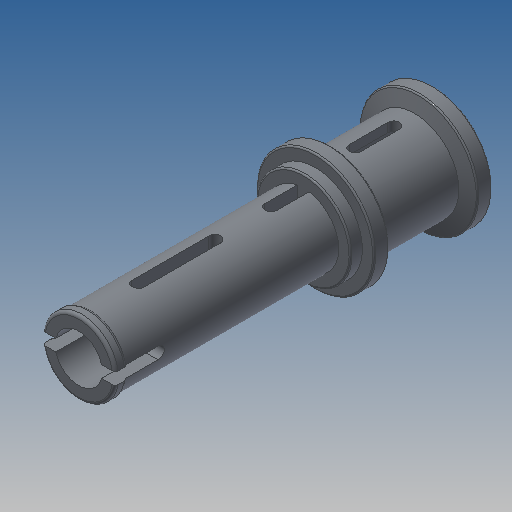
# Autodesk Inventor part: 32054-LtBluishGray
Saved by Autodesk Inventor 2022.2 (Build 262287000, 287)
## iProperties
Created: 2014-06-03
Part Number: 32054-LtBluishGray
Material: ABS Plastic
Document SubType Name: Modeling
Designer: D. Kohfeld
Appearance: LtBluishGray
Density: 1.06 g/cm^3
Mass: 0.348548 g
Surface Area: 8.37071 cm^2
Volume: 0.328818 cm^3
Author: D. Kohfeld
Autodesk Inventor part; units mm, degrees
ref_plane "YZ Plane" through (0, 0, 0) normal (1, 0, 0) x (0, 1, 0)
ref_plane "XZ Plane" through (0, 0, 0) normal (0, 1, 0) x (-1, 0, 0)
ref_plane "XY Plane" through (0, 0, 0) normal (0, 0, 1) x (1, 0, 0)
sketch "Sketch1" plane through (0, 0, 0) normal (0, 1, 0) x (-1, 0, 0)
  line L0 (2.4, 15.2) -> (2.4, 0.8)
  line L1 (3.2, 0.8) -> (2.4, 0.8)
  line L2 (3.2, 0.8) -> (3.2, 0)
  line L3 (3, -6.7321) -> (3, -1.2679)
  line L4 (2.5, 16) -> (2.5, 15.2)
  line L5 (2.5, 16) -> (1.6, 16)
  line L6 (0, -15.68) -> (0, 21.28) projected
  line L7 (2.4, 15.2) -> (2.5, 15.2)
  line L8 (5.28, 0) -> (-3.68, 0) projected
  line L9 (0, -8) -> (4, -8)
  line L10 (4, -8) -> (4, -7)
  line L11 (-0.4, 3) -> (-0.4, 0.8)
  line L12 (0.4, 0.8) -> (0.4, 3)
  arc A0 (0.4, 3) -> (-0.4, 3) centre (0, 3) ccw
  line L13 (-0.4, 12) -> (-0.4, 6.8)
  arc A1 (-0.4, 6.8) -> (0.4, 6.8) centre (0, 6.8) ccw
  line L14 (0.4, 6.8) -> (0.4, 12)
  arc A2 (0.4, 12) -> (-0.4, 12) centre (0, 12) ccw
  line L15 (3.2, 0) -> (4, 0)
  line L16 (4, 0) -> (4, -1)
  line L17 (4, -1) -> (3, -1.2679)
  line L18 (4, -7) -> (3, -6.7321)
  circle A3 centre (0, -8) radius 2.4 construction
  line L19 (-0.4, 0.8) -> (0.4, 0.8)
  line L20 (0.4, -2.7) -> (0.4, -5.3)
  arc A4 (-0.4, -5.3) -> (0.4, -5.3) centre (0, -5.3) ccw
  line L21 (-0.4, -5.3) -> (-0.4, -2.7)
  arc A5 (0.4, -2.7) -> (-0.4, -2.7) centre (0, -2.7) ccw
  line L22 (1.6, 16) -> (1.6, 0)
  line L23 (1.6, 0) -> (0, 0)
  line L24 (0, 0) -> (0, -8)
  point P0 (0.4, -4)
  point P1 (3, -4)
  dimension "d1" = 4.8
  dimension "d2" = 5
  dimension "d6" = 16
  dimension "d7" = 0.8
  dimension "d8" = 6.4
  dimension "d9" = 0.8
  dimension "d14" = 0.8
  dimension "d16" = 6
  dimension "d17" = 0.8
  dimension "d18" = 4
  dimension "d19" = 8
  dimension "d30" = 8
  dimension "d32" = 4.8
  dimension "d33" = 1
  dimension "d35" = 15
  dimension "d36" = 0.6
  dimension "d37" = 3.4
  dimension "d38" = 3.4
  dimension "d46" = 3.2
  constraints: 46 end point, 10 point on circle, 10 tangent, 7 point on line, 6 centre point, 6 parallel, 5 perpendicular, 3 vertical, 2 collinear, 2 equal length, 2 horizontal alignment, 2 midpoint, 1 equal radius, 1 vertical alignment
  measures "d1" diameter of L0 L6
  measures "d2" diameter of L4 L6
  measures "d6" distance between parallel lines of L5 L8
  measures "d7" distance from line of L4.end L5
  measures "d8" diameter of L2 L6
  measures "d9" distance between parallel lines of L1 L8
  measures "d14" diameter of A0
  measures "d17" diameter of A2
  measures "d18" distance from line of A2.centre L5
  measures "d19" distance between parallel lines of L9 L8
  measures "d30" diameter of L10 L6
  measures "d32" diameter of A3
  measures "d33" distance of L9.end L10.end
  measures "d35" angle of L18 L9
  measures "d36" distance edge to line of A3 L3
  measures "d46" diameter of L22 L6
revolve "Revolution1" add sketch "Sketch1" angle 360 about axis through (0, 0, -10) along (0, 0, 1) contours L0 L1 L2 L8 L22 L5 L4 L7 | L8 L16 L17 L3 L18 L10 L9 L6 A4 L20 A5 | A5 L20 A4 L6
fillet "Fillet1" radius 0.2 2 edges at (2.5, 0, 16) (2.5, 0, 15.2)
fillet "Fillet1" radius 0.1 5 edges at (4, 0, 0) (4, 0, -1) (4, 0, -7) (4, 0, -8) (3.2, 0, 0.8)
extrude "Extrusion1" cut sketch "Sketch1" along normal through all both and the other way through all contours A5 L20 A4 L6 | L6 A4 L21 A5 | L19 L11 A0 L6 | L6 A0 L12 L19 | A1 L13 A2 L6 | L6 A2 L14 A1
sketch "Sketch2" plane through (0, 0, 0) normal (1, 0, 0) x (0, 1, 0)
  line L0 (-1.6, 16) -> (1.6, 16) projected
  line L1 (-0.4, 16) -> (0.4, 16)
  line L2 (0.4, 16) -> (0.4, 13)
  line L3 (-0.4, 13) -> (-0.4, 16)
  arc A0 (-0.4, 13) -> (0.4, 13) centre (0, 13) ccw
  point P0 (0, 0)
  point P1 (0, 16)
  dimension "d41" = 0.8
  dimension "d47" = 3.4
  constraints: 6 end point, 2 midpoint, 2 point on circle, 2 tangent, 1 centre point, 1 horizontal, 1 parallel, 1 perpendicular, 1 point on line
  measures "d41" distance between parallel lines of L3 L2
extrude "Extrusion2" cut sketch "Sketch2" along normal through all both and the other way through all
sketch "Sketch3" plane through (0, 0, -8) normal (0, 0, -1) x (-1, 0, 0)
  circle A0 centre (0, 0) radius 3.9 projected
  circle A1 centre (0, 0) radius 2.4 construction
  line L0 (-0.8, 2.2627) -> (-0.8, 0.8)
  line L1 (-0.8, 0.8) -> (-2.2627, 0.8)
  line L2 (-2.2627, -0.8) -> (-0.8, -0.8)
  line L3 (-0.8, -0.8) -> (-0.8, -2.2627)
  line L4 (0.8, -2.2627) -> (0.8, -0.8)
  line L5 (0.8, -0.8) -> (2.2627, -0.8)
  line L6 (2.2627, 0.8) -> (0.8, 0.8)
  line L7 (0.8, 0.8) -> (0.8, 2.2627)
  arc A2 (0.8, 2.2627) -> (-0.8, 2.2627) centre (0, 0) ccw
  arc A3 (-2.2627, 0.8) -> (-2.2627, -0.8) centre (0, 0) ccw
  arc A4 (-0.8, -2.2627) -> (0.8, -2.2627) centre (0, 0) ccw
  arc A5 (2.2627, -0.8) -> (2.2627, 0.8) centre (0, 0) ccw
  dimension "d42" = 4.8
  dimension "d43" = 1.6
  constraints: 16 end point, 8 point on circle, 7 equal length, 4 centre point, 4 perpendicular, 3 parallel, 1 coincident, 1 vertical, 14 other
  measures "d43" distance between parallel lines of L0 L7
extrude "Extrusion3" cut sketch "Sketch3" against normal up to surface (8 mm away) contours A2 L7 L6 A5 L5 L4 A4 L3 L2 A3 L1 L0
equation "\"d1\" = tpd"
equation "\"d2\" = tpcd"
equation "\"d6\" = 2 * lu"
equation "\"d7\" = d9"
equation "\"d8\" = tsd"
equation "\"d9\" = tsl"
equation "\"d14\" = d17"
equation "\"d17\" = tpnw"
equation "\"d19\" = lu"
equation "\"d32\" = kd"
equation "\"d37\" = tpnl"
equation "\"d38\" = d37"
equation "\"d46\" = rd"
equation "\"d27\" = pinf"
equation "\"d28\" = lf"
equation "\"d41\" = tpnw"
equation "\"d47\" = tpnl"
equation "\"d42\" = kd"
equation "\"d43\" = axlet"
equation "\"tpd\" = 4.8"
equation "\"tpcd\" = 5"
equation "\"lu\" = 8"
equation "\"tsd\" = 6.4"
equation "\"tsl\" = 0.8"
equation "\"tpnw\" = 0.8"
equation "\"kd\" = 4.8"
equation "\"tpnl\" = 3.4"
equation "\"rd\" = 3.2"
equation "\"pinf\" = 0.2"
equation "\"lf\" = 0.1"
equation "\"axlet\" = 1.6"
body "Solid2"
